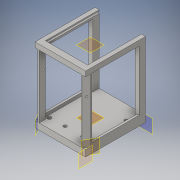
# Autodesk Inventor part: Base
Saved by Autodesk Inventor 2016 (Build 200138000, 138)
## iProperties
Created: 2018-10-15
Part Number: Base
Material: Generic
Document SubType Name: Modeling
Designer: Kyle
Density: 1 g/cm^3
Appearance: Default
Author: Kyle
Autodesk Inventor part; units mm, degrees
note: some values were not read from the file. Chosen so that the rebuilt part matches the saved one: sketch regions of "Extrusion9".
ref_plane "YZ Plane" through (0, 0, 0) normal (1, 0, 0) x (0, 1, 0)
ref_plane "XZ Plane" through (0, 0, 0) normal (0, 1, 0) x (-1, 0, 0)
ref_plane "XY Plane" through (0, 0, 0) normal (0, 0, 1) x (1, 0, 0)
sketch "Sketch1" plane through (0, 0, 0) normal (0, 1, 0) x (-1, 0, 0)
  line L0 (-40, -47.5) -> (40, -47.5)
  line L1 (40, -47.5) -> (40, 47.5)
  line L2 (40, 47.5) -> (-40, 47.5)
  line L3 (-40, 47.5) -> (-40, -47.5)
  line L4 (-40, -47.5) -> (40, 47.5) construction
  line L5 (40, -47.5) -> (-40, 47.5) construction
  line L6 (25.5, 17) -> (28.5, 17)
  line L7 (0, 17.5) -> (0, 19)
  line L8 (0, 0) -> (2.25, 0)
  line L9 (0, 0) -> (0, 17.5)
  line L10 (-27.5, -36.75) -> (-27.5, 38.25)
  line L11 (-27.5, 38.25) -> (28.5, -36.75) construction
  line L12 (28.5, 38.25) -> (-27.5, -36.75) construction
  line L13 (28.5, 38.25) -> (28.5, -36.75)
  line L14 (28.5, 17) -> (28.5, -36.75)
  line L15 (28.5, -36.75) -> (-27.5, -36.75)
  line L16 (0, -31.5) -> (8.5, -31.5)
  line L17 (0, 0) -> (0, -31.5)
  line L18 (0, -31.5) -> (-19.5, -31.5)
  line L19 (-19.5, -31.5) -> (-19.5, -36.75)
  line L20 (-27.5, 38.25) -> (28.5, 38.25)
  line L21 (0, 19) -> (24, 19)
  line L22 (0, 0) -> (0, 31.5)
  line L23 (28.5, -17) -> (28.5, 36.75)
  line L24 (28.5, -38.25) -> (28.5, 36.75)
  line L25 (28.5, -38.25) -> (-27.5, 36.75) construction
  line L26 (-27.5, 36.75) -> (-27.5, -38.25)
  line L27 (-27.5, -38.25) -> (28.5, 36.75) construction
  line L28 (0, 31.5) -> (8.5, 31.5)
  circle A0 centre (8.5, 31.5) radius 2.5
  line L29 (0, 31.5) -> (-19.5, 31.5)
  circle A1 centre (-19.5, 31.5) radius 2.5
  circle A2 centre (-19.5, 31.5) radius 2.5
  line L30 (-19.5, 31.5) -> (-19.5, 36.75)
  line L31 (28.5, 36.75) -> (-27.5, 36.75)
  line L32 (0, 0) -> (0, -17.5)
  line L33 (0, -17.5) -> (0, -19)
  line L34 (25.5, -17) -> (28.5, -17)
  line L35 (0, -19) -> (24, -19)
  line L36 (-27.5, -38.25) -> (28.5, -38.25)
  circle A3 centre (24, -19) radius 2.5
  point P0 (0.5, 0.75)
  point P1 (0.5, -0.75)
  dimension "d0" = 80
  dimension "d1" = 95
  dimension "d5" = 17.5
  dimension "d6" = 8.5
  dimension "d7" = 19.5
  dimension "d8" = 31.5
  dimension "d9" = 24
  dimension "d11" = 2.25
  dimension "d12" = 56
  dimension "d13" = 75
  dimension "d14" = 5.25
  dimension "d15" = 3
  constraints: 74 end point, 14 symmetric about line, 7 horizontal, 6 midpoint, 5 perpendicular, 5 vertical, 4 parallel, 4 point on line, 3 centre point, 1 coincident, 4 other
  measures "d0" distance of L2.end L1.end
  measures "d1" distance of L0.end L1.end
  measures "d5" distance of L17.start L9.end
  measures "d6" distance of L17.end L16.end
  measures "d7" distance of L17.end L18.end
  measures "d8" distance of L17.start L17.end
  measures "d9" distance of L7.end L21.end
  measures "d11" distance of L8.start L8.end
  measures "d12" distance of L14.end L12.end
  measures "d13" distance of L14.end L13.start
  measures "d14" distance of L18.end L19.end
  measures "d15" distance of L6.start L14.start
ref_plane "Work Plane3" through (0, 10, 0) normal (0, 1, 0) x (1, 0, 0)
sketch "Sketch2" plane through (0, 10, 0) normal (0, 1, 0) x (1, 0, 0)
  line L0 (35.5, -47.5) -> (40, -39.7058)
  line L1 (35.5, -47.5) -> (44.5, -47.5) construction
  line L2 (40, -39.7058) -> (35.5, -39.7058)
  line L3 (35.5, -39.7058) -> (35.5, -47.5)
  line L4 (-40, -47.5) -> (40, -47.5) projected
  line L5 (40, -47.5) -> (40, 47.5) projected
  line L6 (40, -37.7058) -> (33.5, -37.7058)
  line L7 (33.5, -37.7058) -> (33.5, -47.5)
  line L8 (33.5, -47.5) -> (35.5, -47.5)
  line L9 (40, -39.7058) -> (40, -37.7058)
  line L10 (0, -47.5) -> (0, 47.5)
  line L11 (-35.5, -47.5) -> (-40, -39.7058)
  line L12 (-35.5, -47.5) -> (-44.5, -47.5) construction
  line L13 (-40, -39.7058) -> (-35.5, -39.7058)
  line L14 (-35.5, -39.7058) -> (-35.5, -47.5)
  line L15 (-40, -37.7058) -> (-33.5, -37.7058)
  line L16 (-33.5, -37.7058) -> (-33.5, -47.5)
  line L17 (-33.5, -47.5) -> (-35.5, -47.5)
  line L18 (-40, -39.7058) -> (-40, -37.7058)
  line L19 (40, 47.5) -> (-40, 47.5) projected
  line L20 (-40, 47.5) -> (-33.5, 47.5)
  line L21 (-33.5, 47.5) -> (-33.5, 37.5)
  line L22 (-33.5, 37.5) -> (-40, 37.5)
  line L23 (-40, 37.5) -> (-40, 47.5)
  line L24 (40, 47.5) -> (33.5, 47.5)
  line L25 (33.5, 47.5) -> (33.5, 37.5)
  line L26 (33.5, 37.5) -> (40, 37.5)
  line L27 (40, 37.5) -> (40, 47.5)
  point P0 (0, 0)
  dimension "d18" = 9
  dimension "d19" = 60
  dimension "d20" = 2
  dimension "d21" = 9.7942
  dimension "d22" = 6.5
  dimension "d23" = 6.5
  dimension "d24" = 10
  dimension "d25" = 6.5
  dimension "d26" = 10
  constraints: 50 end point, 7 symmetric about line, 4 horizontal, 4 parallel, 4 perpendicular, 4 point on line, 2 collinear, 1 equal length, 1 midpoint, 1 vertical
  measures "d18" distance of L0.start L0.end
  measures "d19" angle of L1 L0
  measures "d20" distance between parallel lines of L3 L7
  measures "d21" distance of L6.end L7.end
  measures "d22" distance of L6.start L6.end
  measures "d23" distance of L21.end L22.end
  measures "d24" distance of L20.end L21.end
  measures "d25" distance of L26.end L25.end
  measures "d26" distance of L25.end L24.end
extrude "Extrusion2" add sketch "Sketch2" along normal blind 100 contours L3 L2 L0 | L4 L7 L6 L5 L2 L3 | L26 L25 L19 L5 | L14 L13 L18 L15 L16 L4 | L11 L13 L14 | L21 L22 L23 L19
ref_plane "Work Plane2" through (0, 10, 0) normal (0, 1, 0) x (1, 0, 0)
sketch "Sketch3" plane through (0, 10, 0) normal (0, 1, 0) x (1, 0, 0)
  line L0 (-40, 37.5) -> (-40, -37.7058) projected
  line L1 (-33.5, 37.5) -> (-40, 37.5) projected
  line L2 (-40, -37.7058) -> (-36.75, -37.7058)
  line L3 (-36.75, -37.7058) -> (-36.75, 37.5)
  line L4 (-36.75, 37.5) -> (-40, 37.5)
  line L5 (-40, 37.5) -> (-40, -37.7058)
  line L6 (33.5, 37.5) -> (40, 37.5) projected
  line L7 (40, -37.7058) -> (33.5, -37.7058) projected
  line L8 (40, 37.5) -> (36.75, 37.5)
  line L9 (36.75, 37.5) -> (36.75, -37.7058)
  line L10 (36.75, -37.7058) -> (40, -37.7058)
  line L11 (40, -37.7058) -> (40, 37.5)
  point P0 (0, 0)
  constraints: 16 end point, 4 parallel, 2 horizontal, 2 midpoint, 2 perpendicular
extrude "Extrusion3" add sketch "Sketch3" along normal blind 5
ref_plane "Work Plane4" through (0, 110, 0) normal (0, 1, 0) x (1, 0, 0)
sketch "Sketch4" plane through (0, 110, 0) normal (0, 1, 0) x (1, 0, 0)
  line L0 (-33.5, 47.5) -> (-40, 47.5) projected
  line L1 (-40, -47.5) -> (40, -47.5) projected
  line L2 (-40, 47.5) -> (-33.5, 47.5)
  line L3 (-33.5, 47.5) -> (-33.5, -47.5)
  line L4 (-33.5, -47.5) -> (-40, -47.5)
  line L5 (-40, -47.5) -> (-40, 47.5)
  line L6 (40, 37.5) -> (40, 47.5) projected
  line L7 (40, 47.5) -> (33.5, 47.5)
  line L8 (33.5, 47.5) -> (33.5, -47.5)
  line L9 (33.5, -47.5) -> (40, -47.5)
  line L10 (40, -47.5) -> (40, 47.5)
  line L11 (40, -37.7058) -> (33.5, -37.7058) projected
  line L12 (33.5, -37.7058) -> (-33.5, -37.7058)
  line L13 (-33.5, -37.7058) -> (-33.5, -47.5)
  line L14 (-33.5, -47.5) -> (33.5, -47.5)
  line L15 (33.5, -47.5) -> (33.5, -37.7058)
  point P0 (0, 0)
  constraints: 24 end point, 6 parallel, 3 horizontal, 3 perpendicular, 2 point on line
extrude "Extrusion4" add sketch "Sketch4" along normal blind 8
ref_plane "Work Plane8" through (40, 0, -47.5) normal (0, 0, -1) x (-1, 0, 0)
sketch "Sketch5" plane through (40, 0, -47.5) normal (0, 0, -1) x (-1, 0, 0)
  line L0 (73.5, 110) -> (6.5, 110) projected
  line L1 (6.5, 110) -> (6.5, 113)
  line L2 (6.5, 10) -> (6.5, 118) projected
  line L3 (6.5, 113) -> (3.25, 113)
  line L4 (3.25, 113) -> (3.25, 116)
  line L5 (3.25, 116) -> (6.5, 116)
  line L6 (6.5, 116) -> (6.5, 113)
  line L7 (73.5, 10) -> (73.5, 118) projected
  line L8 (6.5, 116) -> (73.5, 116)
  line L9 (73.5, 116) -> (73.5, 113)
  line L10 (73.5, 113) -> (6.5, 113)
  line L11 (6.5, 113) -> (6.5, 116)
  line L12 (73.5, 113) -> (76.75, 113)
  line L13 (76.75, 113) -> (76.75, 116)
  line L14 (76.75, 116) -> (73.5, 116)
  line L15 (73.5, 116) -> (73.5, 113)
  point P0 (40, 0)
  dimension "d33" = 3
  dimension "d34" = 3
  dimension "d35" = 3.25
  dimension "d36" = 3.25
  constraints: 26 end point, 5 perpendicular, 4 parallel, 4 point on line, 2 horizontal, 1 collinear
  measures "d33" distance of L0.end L1.end
  measures "d34" distance of L3.end L4.end
  measures "d35" distance of L14.end L13.end
  measures "d36" distance of L4.end L5.end
extrude "Extrusion5" cut sketch "Sketch5" against normal blind 90.206 contours L10 L2 L8 L7 | L7 L14 L13 L12 | L3 L4 L5 L2
ref_plane "Work Plane7" through (40, 10, 39.7058) normal (0.8660254, 0, 0.5) x (0.5, 0, -0.8660254)
sketch "Sketch6" plane through (40, 10, 39.7058) normal (0.8660254, 0, 0.5) x (0.5, 0, -0.8660254)
  line L0 (-9, 0) -> (-9, 100) projected
  line L1 (0, 0) -> (-9, 0) projected
  line L2 (-9, 100) -> (0, 100)
  line L3 (0, 100) -> (0, 0)
  line L4 (0, 0) -> (-9, 0)
  line L5 (-9, 0) -> (-9, 100)
  line L6 (0, 100) -> (0, 70)
  line L7 (0, 0) -> (0, 100) projected
  line L8 (0, 70) -> (-4.5, 70)
  circle A0 centre (-4.5, 70) radius 1.5
  point P0 (14.3862, -10)
  dimension "d39" = 30
  dimension "d40" = 3
  constraints: 12 end point, 2 parallel, 2 perpendicular, 1 centre point, 1 coincident, 1 horizontal, 1 point on line
  measures "d39" distance of L2.end L6.end
  measures "d40" diameter of A0
extrude "Extrusion6" cut sketch "Sketch6" against normal blind 6 contours A0
ref_plane "Work Plane6" through (-35.5, 10, 47.5) normal (-0.8660254, 0, 0.5) x (0.5, 0, 0.8660254)
sketch "Sketch7" plane through (-35.5, 10, 47.5) normal (-0.8660254, 0, 0.5) x (0.5, 0, 0.8660254)
  line L0 (-9, 0) -> (-9, 100) projected
  line L1 (0, 0) -> (0, 100) projected
  line L2 (-9, 100) -> (0, 100)
  line L3 (0, 100) -> (0, 0)
  line L4 (0, 0) -> (-9, 0)
  line L5 (-9, 0) -> (-9, 100)
  line L6 (-9, 100) -> (-9, 70)
  line L7 (-9, 70) -> (-4.5, 70)
  circle A0 centre (-4.5, 70) radius 1.5
  point P0 (-23.3862, -10)
  dimension "d43" = 30
  dimension "d44" = 3
  constraints: 12 end point, 2 parallel, 2 perpendicular, 1 centre point, 1 coincident, 1 horizontal, 1 point on line
  measures "d43" distance of L0.end L6.end
  measures "d44" diameter of A0
extrude "Extrusion7" cut sketch "Sketch7" against normal blind 6 contours A0
ref_plane "Work Plane5" through (40, 0, 47.5) normal (1, 0, 0) x (0, 0, -1)
sketch "Sketch8" plane through (40, 0, 47.5) normal (1, 0, 0) x (0, 0, -1)
  line L0 (85, 110) -> (9.7942, 110) projected
  line L1 (85, 110) -> (95, 110)
  line L2 (95, 110) -> (95, 80)
  line L3 (95, 80) -> (85, 80)
  line L4 (85, 80) -> (85, 110)
  circle A0 centre (90, 80) radius 1.5
  point P0 (47.5, 0)
  dimension "d47" = 10
  dimension "d48" = 30
  dimension "d49" = 3
  constraints: 8 end point, 2 parallel, 1 centre point, 1 horizontal, 1 midpoint, 1 perpendicular
  measures "d47" distance of L2.end L3.end
  measures "d48" distance of L1.end L2.end
  measures "d49" diameter of A0
extrude "Extrusion8" [suppressed]
ref_plane "Work Plane1" through (0, 0, 0) normal (0, -1, 0) x (1, 0, 0)
sketch "Sketch9" plane through (0, 0, 0) normal (0, -1, 0) x (1, 0, 0)
  line L0 (40, 47.5) -> (40, 39.7058) projected
  line L1 (40, 47.5) -> (25, 47.5)
  line L2 (25, 47.5) -> (25, -10)
  line L3 (25, -10) -> (40, -10)
  line L4 (40, -10) -> (40, 47.5)
  line L5 (-40, 47.5) -> (-35.5, 47.5) projected
  line L6 (-40, 47.5) -> (-25, 47.5)
  line L7 (-25, 47.5) -> (-25, -10)
  line L8 (-25, -10) -> (-40, -10)
  line L9 (-40, -10) -> (-40, 47.5)
  line L10 (-40, 47.5) -> (40, 47.5) projected
  line L11 (-40, 47.5) -> (-32.5, 47.5)
  line L12 (-33.5, 47.5) -> (-33.5, 37.7058) projected
  line L13 (-40, 47.5) -> (-33.5, 47.5)
  line L14 (-33.5, 47.5) -> (-29, 47.5)
  line L15 (-40, 47.5) -> (-32.5, 47.5)
  line L16 (-32.5, 47.5) -> (-32.5, 32.5)
  circle A0 centre (-32.5, 32.5) radius 3
  line L17 (-32.5, -10) -> (-32.5, -25)
  circle A1 centre (-32.5, -25) radius 3
  line L18 (32.5, 47.5) -> (32.5, 32.5)
  line L19 (32.5, -10) -> (32.5, -25)
  circle A2 centre (32.5, -25) radius 3
  circle A3 centre (32.5, 32.5) radius 3
  point P0 (0, 0)
  dimension "d52" = 15
  dimension "d53" = 57.5
  dimension "d54" = 15
  dimension "d55" = 57.5
  dimension "d61" = 7.5
  dimension "d62" = 15
  dimension "d63" = 6
  dimension "d64" = 15
  dimension "d65" = 6
  dimension "d66" = 15
  dimension "d67" = 15
  dimension "d68" = 6
  dimension "d69" = 6
  constraints: 32 end point, 4 centre point, 4 coincident, 4 parallel, 4 perpendicular, 3 point on line, 2 collinear, 2 horizontal, 2 midpoint, 2 vertical
  measures "d52" distance of L3.end L2.end
  measures "d53" distance of L2.end L1.end
  measures "d54" distance of L7.end L8.end
  measures "d55" distance of L6.end L7.end
  measures "d61" distance of L5.start L11.end
  measures "d62" distance of L11.end L16.end
  measures "d63" diameter of A0
  measures "d64" distance of L17.start L17.end
  measures "d65" diameter of A1
  measures "d66" distance of L18.start L18.end
  measures "d67" distance of L19.start L19.end
  measures "d68" diameter of A2
  measures "d69" diameter of A3
extrude "Extrusion9" add sketch "Sketch1" along normal blind 10 contours L3 L2 L1 L0 | L9 L17 L18 L19 L15 L10 L31 L30 A1 L29 L22 L7 | L7 L22 L29 A1 L30 L31 L13 L34 A3 L35 L17 L9 | L35 A3 L34 L13 L15 L19 L18 L17 | L31 L10 L20 L13 | L15 L24 L36 L26
extrude "Extrusion11" cut sketch "Sketch9" against normal up to surface (10 mm away) contours A0 | A1 | A2 | A3
equation "\"d72\" = d68"
body "Solid1"
